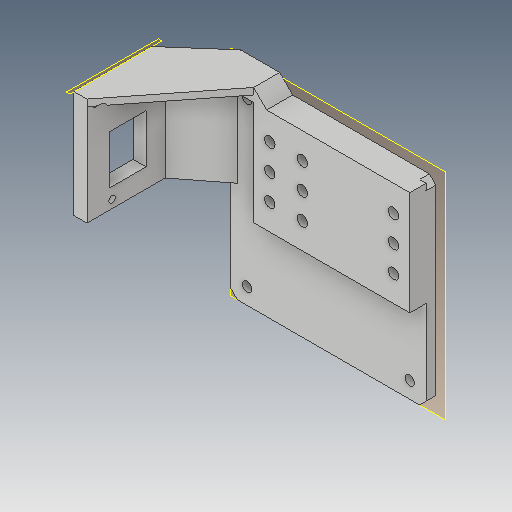
# Autodesk Inventor part: cellSTORM_inverted_Laser_left
Saved by Autodesk Inventor 2019.4 (Build 234330000, 330)
## iProperties
Created: 2020-11-05
Part Number: cellSTORM_inverted_Laser_left
Material: Generic
Document SubType Name: Modeling
Designer: diederichbenedict
Density: 1 g/cm^3
Appearance: Default
Author: diederichbenedict
Autodesk Inventor part; units mm, degrees
ref_plane "Work Plane1" through (0, 0, 0) normal (0, 0, 1) x (1, 0, 0)
sketch "Sketch1" plane through (0, 0, 0) normal (0, 0, 1) x (1, 0, 0)
  circle A0 centre (0, 25) radius 1.95 construction
  circle A1 centre (-25, 0) radius 1.95 construction
  circle A2 centre (-25, -25) radius 1.95 construction
  circle A3 centre (25, 25) radius 1.95 construction
  circle A4 centre (25, -25) radius 1.95 construction
  circle A5 centre (-25, 25) radius 1.95 construction
  circle A6 centre (25, 0) radius 1.95 construction
  circle A7 centre (0, -25) radius 1.95 construction
  line L0 (-28, 30) -> (-30, 28) projected
  line L1 (-30, 28) -> (-30, -28) projected
  line L2 (-30, -28) -> (-28, -30) projected
  line L3 (-28, -30) -> (28, -30) projected
  line L4 (28, -30) -> (30, -28) projected
  line L5 (30, -28) -> (30, 28) projected
  line L6 (30, 28) -> (28, 30) projected
  line L7 (28, 30) -> (-28, 30) projected
  circle A8 centre (25, 25) radius 1.45
  circle A9 centre (25, -25) radius 1.45
  circle A10 centre (-25, -25) radius 1.45
  circle A11 centre (-25, 25) radius 1.45
  circle A12 centre (0, 25) radius 1.95 projected
  circle A13 centre (-25, 0) radius 1.95 projected
  circle A14 centre (-25, -25) radius 1.95 projected
  circle A15 centre (25, 25) radius 1.95 projected
  circle A16 centre (25, -25) radius 1.95 projected
  circle A17 centre (-25, 25) radius 1.95 projected
  circle A18 centre (25, 0) radius 1.95 projected
  circle A19 centre (0, -25) radius 1.95 projected
  line L8 (-28, 30) -> (-30, 28) projected
  line L9 (-30, 28) -> (-30, -28) projected
  line L10 (-30, -28) -> (-28, -30) projected
  line L11 (-28, -30) -> (28, -30) projected
  line L12 (28, -30) -> (30, -28) projected
  line L13 (30, -28) -> (30, 28) projected
  line L14 (30, 28) -> (28, 30) projected
  line L15 (28, 30) -> (-28, 30) projected
  line L16 (-44.5, 28.8555) -> (-44.5, 2)
  line L17 (-44.5, 34) -> (-45.5, 34)
  line L18 (-45.5, 1) -> (-44.5, 1)
  line L19 (-44.5, 34) -> (-30, 34)
  line L20 (-30, 34) -> (-30, 1)
  line L21 (-30, 1) -> (-44.5, 1)
  line L22 (-44.5, 1) -> (-44.5, 34)
  line L23 (-30, 34) -> (-26, 30)
  line L24 (-30, 34) -> (-24.3431, 34) construction
  point P0 (0, 0)
  dimension "d0" = 2.9
  dimension "d1" = 2.9
  dimension "d2" = 2.9
  dimension "d3" = 2.9
  dimension "d6" = 45
  constraints: 18 end point, 4 centre point, 4 horizontal, 3 coincident, 2 parallel, 2 point on line, 1 equal length, 1 perpendicular, 1 vertical, 6 other
  measures "d0" diameter of A8
  measures "d1" diameter of A9
  measures "d2" diameter of A10
  measures "d3" diameter of A11
  measures "d6" angle of L23 L24
ref_plane "Work Plane2" through (-18, -2, 8) normal (0, 0, -1) x (0, 1, 0)
extrude "Extrusion1" add sketch "Sketch1" along normal blind 3 contours L7 L6 L5 L4 L3 L2 L1 L0 | A12 | A13 | A14 | A15 | A16 | A17 | A18 | A19
sketch "Sketch2" plane through (0, 0, 3) normal (0, 0, 1) x (1, 0, 0)
  circle A0 centre (-3, 22) radius 1.4 projected
  circle A1 centre (-3, 14) radius 1.4 projected
  circle A2 centre (-13, 6) radius 1.4 projected
  circle A3 centre (-13, 14) radius 1.4 projected
  circle A4 centre (25, 14) radius 1.4 projected
  circle A5 centre (25, 6) radius 1.4 projected
  circle A6 centre (-13, 22) radius 1.4 projected
  circle A7 centre (-3, 6) radius 1.4 projected
  circle A8 centre (25, 22) radius 1.4 projected
  line L0 (30, -2) -> (30, 30) projected
  line L1 (30, -2) -> (-18, -2) projected
  line L2 (-18, 30) -> (-18, -2) projected
  line L3 (30, 30) -> (-18, 30) projected
  point P0 (0, 0)
ref_plane "Work Plane3" through (-18, -2, 8) normal (0, 0, -1) x (0, 1, 0)
extrude "Extrusion2" add sketch "Sketch2" along normal up to surface (5 mm away)
sketch "Sketch3" plane through (0, 0, 0) normal (0, 0, -1) x (-1, 0, 0)
  circle A0 centre (-25, 22) radius 1.4 projected
  circle A1 centre (3, 6) radius 1.4 projected
  circle A2 centre (13, 22) radius 1.4 projected
  circle A3 centre (-25, 6) radius 1.4 projected
  circle A4 centre (-25, 14) radius 1.4 projected
  circle A5 centre (13, 14) radius 1.4 projected
  circle A6 centre (13, 6) radius 1.4 projected
  circle A7 centre (3, 14) radius 1.4 projected
  circle A8 centre (3, 22) radius 1.4 projected
  line L0 (18, -2) -> (-30, -2) projected
  line L1 (-30, -2) -> (-30, 30) projected
  line L2 (-30, 30) -> (18, 30) projected
  line L3 (18, 30) -> (18, -2) projected
  point P0 (0, 0)
hole "Hole2" at (-13, 6, 0) at (-13, 14, 0) at (-13, 22, 0) at (-3, 22, 0) at (-3, 14, 0) at (-3, 6, 0) at (25, 6, 0) at (25, 14, 0) at (25, 22, 0) direction (0, 0, 1) diameter 3.2 depth 20 tip angle 118 counterbore diameter 5 counterbore depth 4
ref_plane "Work Plane4" through (-44.5, 34, 36.7) normal (0, 1, 0) x (0, 0, -1)
sketch "Sketch5" plane through (-44.5, 34, 36.7) normal (0, 1, 0) x (0, 0, -1)
  line L0 (36.7, -72.5) -> (36.7, -16.5) projected
  line L1 (36.7, -16.5) -> (33.7, -16.5) projected
  line L2 (33.7, -26.5) -> (33.7, -16.5) projected
  line L3 (33.7, -26.5) -> (28.7, -26.5) projected
  line L4 (28.7, -74.5) -> (28.7, -26.5) projected
  line L5 (33.7, -74.5) -> (28.7, -74.5) projected
  line L6 (33.7, -74.5) -> (33.7, -72.5) projected
  line L7 (36.7, -72.5) -> (33.7, -72.5) projected
  line L8 (25.7, 0) -> (0, 0) projected
  line L9 (25.7, 0) -> (25.7, 1) projected
  line L10 (0, 1) -> (25.7, 1) projected
  line L11 (0, 0) -> (0, 1) projected
  line L12 (0, 0) -> (24, 0)
  line L13 (24, 0) -> (24, -4)
  line L14 (24, -4) -> (0, -4)
  line L15 (0, -4) -> (0, 0)
  line L16 (24, -4) -> (33.7, -16.5)
  line L17 (36.7, -16.5) -> (36.7, -14.5) projected
  line L18 (36.7, -14.5) -> (36.7, -16.5) projected
  line L19 (24, 0) -> (36.7, -14.5)
  line L20 (36.7, -16.5) -> (33.7, -16.5) projected
  line L21 (36.7, -14.5) -> (36.7, -16.5)
  point P0 (36.7, -44.5)
  dimension "d23" = 24
  dimension "d24" = 4
  constraints: 14 end point, 2 parallel, 2 perpendicular, 1 horizontal
  measures "d23" distance of L13.end L14.end
  measures "d24" distance of L12.end L13.end
ref_plane "Work Plane5" through (-45.5, 1, 28.397) normal (0, -1, 0) x (1, 0, 0)
extrude "Extrusion3" add sketch "Sketch5" against normal up to surface (33 mm away) contours L1 L16 L13 L19 L17 | L14 L15 L8 L13
sketch "Sketch6" plane through (-44.5, 34, 36.7) normal (0, 1, 0) x (1, 0, 0)
  line L0 (0, 0) -> (0, 24) projected
  line L1 (4, 0) -> (0, 0) projected
  line L2 (4, 24) -> (4, 0) projected
  line L3 (16.5, 33.7) -> (4, 24) projected
  line L4 (26.5, 33.7) -> (26.5, 28.7) projected
  line L5 (26.5, 28.7) -> (4, 0)
  line L6 (0, 24) -> (14.5, 36.7) projected
  line L7 (14.5, 36.7) -> (16.5, 36.7) projected
  line L8 (16.5, 36.7) -> (16.5, 33.7) projected
  line L9 (26.5, 33.7) -> (26.5, 28.7) projected
  line L10 (16.5, 36.7) -> (26.5, 36.7)
  line L11 (26.5, 36.7) -> (26.5, 28.7)
  line L12 (26.5, 28.7) -> (16.5, 28.7)
  line L13 (16.5, 28.7) -> (16.5, 36.7)
  point P0 (44.5, 36.7)
  constraints: 10 end point, 2 parallel, 1 horizontal, 1 perpendicular
extrude "Extrusion4" add sketch "Sketch6" against normal blind 2
sketch "Sketch7" plane through (-44.5, 1, 36.7) normal (-1, 0, 0) x (0, 0, 1)
  circle A0 centre (-7.7, 2.5) radius 1 projected
  circle A1 centre (-2.7, 30.5) radius 1 projected
  circle A2 centre (-23.2, 24) radius 1 projected
  circle A3 centre (-12.7, 13) radius 2.6486 projected
  line L0 (-18.1576, 5.885) -> (-7.0605, 5.885)
  line L1 (-7.0605, 5.885) -> (-7.0605, 20.8532)
  line L2 (-7.0605, 20.8532) -> (-18.1576, 20.8532)
  line L3 (-18.1576, 20.8532) -> (-18.1576, 5.885)
  point P0 (-36.7, -1)
  constraints: 8 end point, 2 parallel, 1 horizontal, 1 perpendicular
extrude "Extrusion5" cut sketch "Sketch7" against normal through all contours A0 | A1 | A2 | A3 | L3 L2 L1 L0
sketch "Sketch8" plane through (0, 0, 0) normal (0, 0, -1) x (-1, 0, 0)
  line L0 (28, 32) -> (28, 30) projected
  line L1 (-28, 30) -> (28, 30) projected
  line L2 (-30, 28) -> (-28, 30) projected
  line L3 (-30, -28) -> (-30, 28) projected
  line L4 (-28, -30) -> (-30, -28) projected
  line L5 (28, -30) -> (-28, -30) projected
  line L6 (30, -28) -> (28, -30) projected
  line L7 (30, 1) -> (30, -28) projected
  line L8 (30, 34) -> (30, 1) projected
  line L9 (30, 34) -> (18, 34) projected
  line L10 (18, 34) -> (18, 32) projected
  line L11 (28, 32) -> (18, 32) projected
  circle A0 centre (25, -25) radius 1.45 projected
  arc A1 (-26.2035, 24.1913) -> (-23.7965, 24.1913) centre (-25, 22) ccw projected
  arc A2 (-23.7965, 24.1913) -> (-26.2035, 24.1913) centre (-25, 25) ccw projected
  circle A3 centre (-25, -25) radius 1.45 projected
  circle A4 centre (25, 25) radius 1.45 projected
  circle A5 centre (-25, 6) radius 2.5 projected
  circle A6 centre (3, 14) radius 2.5 projected
  circle A7 centre (13, 22) radius 2.5 projected
  circle A8 centre (13, 6) radius 2.5 projected
  circle A9 centre (13, 14) radius 2.5 projected
  circle A10 centre (3, 22) radius 2.5 projected
  circle A11 centre (3, 6) radius 2.5 projected
  circle A12 centre (-25, 14) radius 2.5 projected
  line L12 (18, 34) -> (18, 32) projected
  line L13 (18, 34) -> (14, 30)
  line L14 (18, 34) -> (23.6569, 34) construction
  line L15 (-28, 30) -> (28, 30) projected
  point P0 (0, 0)
  dimension "d31" = 135
  constraints: 4 end point, 2 point on line, 1 equal length, 1 horizontal
  measures "d31" angle of L13 L14
extrude "Extrusion6" add sketch "Sketch8" against normal up to surface (8 mm away) contours L0 L1 L13 L10 L11
body "Solid1"
